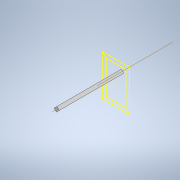
# Autodesk Inventor part: Leg
Saved by Autodesk Inventor 2022 (Build 260153000, 153)
## iProperties
Created: 2021-12-19
Part Number: Leg
Material: Generic
Document SubType Name: Modeling
Designer: dangl
Density: 1 g/cm^3
Appearance: Default
Author: dangl
Autodesk Inventor part; units mm, degrees
ref_plane "YZ Plane" through (0, 0, 0) normal (1, 0, 0) x (0, 1, 0)
ref_plane "XZ Plane" through (0, 0, 0) normal (0, 1, 0) x (-1, 0, 0)
ref_plane "XY Plane" through (0, 0, 0) normal (0, 0, 1) x (1, 0, 0)
sketch "Sketch1" plane through (0, 0, 0) normal (0, 0, 1) x (1, 0, 0)
  line L0 (3.6144, -6.1144) -> (3.6144, 6.1144) projected
  line L1 (3.6144, 6.1144) -> (-3.6144, 6.1144) projected
  line L2 (-3.6144, 6.1144) -> (-3.6144, -6.1144) projected
  line L3 (-3.6144, -6.1144) -> (3.6144, -6.1144) projected
  line L4 (5, -7.5) -> (3.6144, -6.1144) projected
  line L5 (5, 7.5) -> (5, -7.5) projected
  line L6 (3.6144, 6.1144) -> (5, 7.5) projected
  line L7 (3.6144, -6.1144) -> (3.6144, 6.1144) projected
  line L8 (3.6144, 6.1144) -> (5, 7.5) projected
  line L9 (-5, 7.5) -> (5, 7.5) projected
  line L10 (-5, 7.5) -> (-3.6144, 6.1144) projected
  line L11 (3.6144, 6.1144) -> (-3.6144, 6.1144) projected
  line L12 (-3.6144, -6.1144) -> (-5, -7.5) projected
  line L13 (-3.6144, 6.1144) -> (-3.6144, -6.1144) projected
  line L14 (-5, 7.5) -> (-3.6144, 6.1144) projected
  line L15 (-5, -7.5) -> (-5, 7.5) projected
  line L16 (5, -7.5) -> (3.6144, -6.1144) projected
  line L17 (-3.6144, -6.1144) -> (3.6144, -6.1144) projected
  line L18 (-3.6144, -6.1144) -> (-5, -7.5) projected
  line L19 (5, -7.5) -> (-5, -7.5) projected
  point P0 (0, 0)
ref_plane "Work Plane2" through (3.6144, 6.1144, 0) normal (0.7071068, -0.7071068, 0) x (0.7071068, 0.7071068, 0)
ref_plane "Work Plane1" through (0, 0, 0) normal (0, 0, 1) x (1, 0, 0)
sketch "Sketch2" plane through (3.6144, 6.1144, 0) normal (0.7071068, -0.7071068, 0) x (0.7071068, 0.7071068, 0)
  line L0 (-0.9695, 0.5) -> (3.7914, 27.5)
  line L1 (3.7914, 27.5) -> (2.2914, 27.5)
  line L2 (2.2914, 27.5) -> (-3.9695, 0.5)
  line L3 (-3.9695, 0.5) -> (-0.9695, 0.5)
  point P0 (-6.8792, 0)
  dimension "d1" = 1.5
  dimension "d2" = 0.5
  dimension "d3" = 3
  dimension "d4" = 27
  dimension "d5" = 80
  constraints: 8 end point, 1 horizontal, 1 parallel
  measures "d1" distance of L0.end L1.end
  measures "d2" distance from line of point (-6.879, 0) L3
  measures "d3" distance of L2.end L0.start
  measures "d4" distance between parallel lines of L1 L3
  measures "d5" angle of L1 L0
extrude "Extrusion1" add sketch "Sketch2" along normal mid plane 1.2
body "Solid1"
